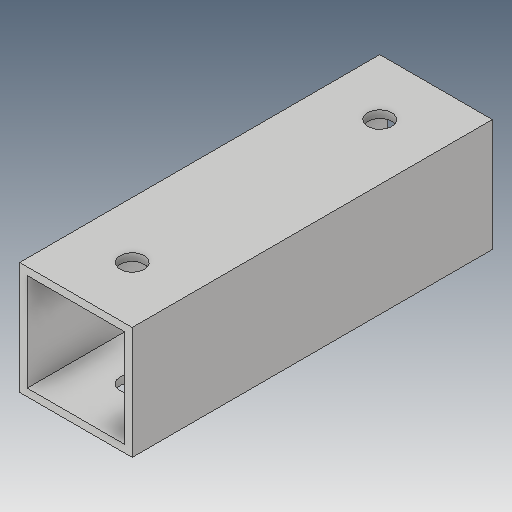
# Autodesk Inventor part: SlideHOLDsq
Saved by Autodesk Inventor 2019.4 (Build 234330000, 330)
## iProperties
Created: 2019-07-02
Part Number: SlideHOLDsq
Material: Generic
Document SubType Name: Modeling
Designer: AzLIer
Density: 1 g/cm^3
Appearance: Default
Author: AzLIer
Autodesk Inventor part; units mm, degrees
ref_plane "YZ Plane" through (0, 0, 0) normal (1, 0, 0) x (0, 1, 0)
ref_plane "XZ Plane" through (0, 0, 0) normal (0, 1, 0) x (-1, 0, 0)
ref_plane "XY Plane" through (0, 0, 0) normal (0, 0, 1) x (1, 0, 0)
sketch "スケッチ1" plane through (0, 0, 0) normal (0, 0, 1) x (1, 0, 0)
  line L0 (-7.5, -7.5) -> (7.5, -7.5)
  line L1 (7.5, -7.5) -> (7.5, 7.5)
  line L2 (7.5, 7.5) -> (-7.5, 7.5)
  line L3 (-7.5, 7.5) -> (-7.5, -7.5)
  line L4 (-7.5, -7.5) -> (7.5, 7.5) construction
  line L5 (7.5, -7.5) -> (-7.5, 7.5) construction
  point P0 (0, 0)
  dimension "d0" = 15
  dimension "d1" = 15
  constraints: 12 end point, 2 midpoint, 2 parallel, 1 horizontal, 1 perpendicular
  measures "d0" distance of L2.end L1.end
  measures "d1" distance of L1.end L0.end
extrude "押し出し1" add sketch "スケッチ1" along normal blind 48
shell "シェル1" thickness 1 removed faces 2 at (-2.5, 2.5, 0) at (-2.5, 2.5, 48)
sketch "スケッチ2" plane through (-7.5, -7.5, 0) normal (0, -1, 0) x (1, 0, 0)
  line L0 (0, 0) -> (15, 0) projected
  point P0 (7.5, 0)
  point P1 (7.5, 7.5)
  point P2 (7.5, 0)
  point P3 (7.5, 40.5)
  point P4 (7.5, 0)
  dimension "d5" = 7.5
  dimension "d13" = 33
  constraints: 2 midpoint, 2 vertical alignment
  measures "d5" distance from line of L0 point (7.5, 7.5)
  measures "d13" distance of point (7.5, 7.5) point (7.5, 40.5)
hole "穴1" at (0, -7.5, 7.5) at (0, -7.5, 40.5) direction (0, 1, 0) diameter 3.2 end through all
